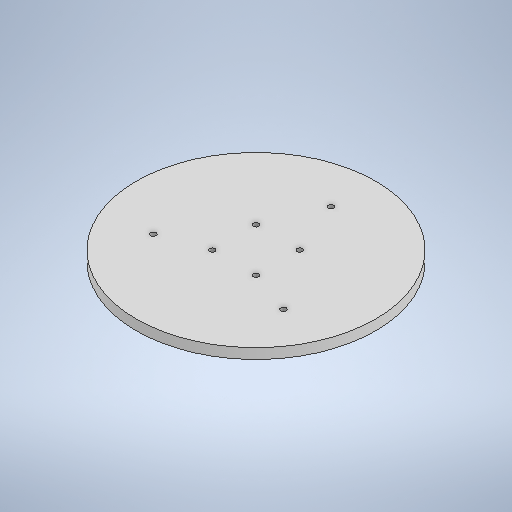
# Autodesk Inventor part: Verbindungsplatte_Staender
Saved by Autodesk Inventor 2025.2 (Build 292293000, 293)
## iProperties
Created: 2025-06-23
Part Number: Verbindungsplatte_Staender
Material: Generisch
Document SubType Name: Modeling
Designer: Jakob
Density: 1 g/cm^3
Appearance: Vorgabe
Author: Jakob
Autodesk Inventor part; units mm, degrees
ref_plane "YZ Plane" through (0, 0, 0) normal (1, 0, 0) x (0, 1, 0)
ref_plane "XZ Plane" through (0, 0, 0) normal (0, 1, 0) x (-1, 0, 0)
ref_plane "XY Plane" through (0, 0, 0) normal (0, 0, 1) x (1, 0, 0)
sketch "Skizze1" plane through (0, 0, 0) normal (0, 0, 1) x (1, 0, 0)
  circle A0 centre (0, 0) radius 175
  dimension "d0" = 350
  constraints: 1 centre point, 1 coincident
  measures "d0" diameter of A0
extrude "Extrusion1" add sketch "Skizze1" against normal blind 15
sketch "Skizze2" plane through (0, 0, 0) normal (0, 0, 1) x (1, 0, 0)
  line L0 (-32, 32) -> (32, 32)
  line L1 (32, 32) -> (32, -32)
  line L2 (32, -32) -> (-32, -32)
  line L3 (-32, -32) -> (-32, 32)
  line L4 (-32, 32) -> (32, -32) construction
  line L5 (32, 32) -> (-32, -32) construction
  circle A0 centre (0, 0) radius 110
  line L6 (0, -245) -> (0, 245) projected
  point P0 (0, 110)
  point P1 (-95.2628, -55)
  point P2 (95.2628, -55)
  dimension "d3" = 64
  dimension "d4" = 64
  dimension "d5" = 220
  constraints: 12 end point, 5 coincident, 3 point on circle, 2 midpoint, 2 parallel, 1 centre point, 1 horizontal, 1 perpendicular
  measures "d3" distance of L0.start L0.end
  measures "d4" distance of L0.end L1.end
  measures "d5" diameter of A0
hole "Bohrung1" at (32, 32, 0) at (-32, 32, 0) at (-32, -32, 0) at (32, -32, 0) at (0, 110, 0) at (-95.2628, -55, 0) at (95.2628, -55, 0) direction (0, 0, -1) diameter 8 end through all
